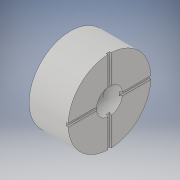
# Autodesk Inventor part: parabol_mirror_1_grooves
Saved by Autodesk Inventor 2019 (Build 230136000, 136)
## iProperties
Created: 2019-08-16
Part Number: parabol_mirror_1_grooves
Material: Generic
Document SubType Name: Modeling
Designer: CyrilLAPLANE
Density: 1 g/cm^3
Appearance: Default
Author: CyrilLAPLANE
Autodesk Inventor part; units mm, degrees
ref_plane "YZ Plane" through (0, 0, 0) normal (1, 0, 0) x (0, 1, 0)
ref_plane "XZ Plane" through (0, 0, 0) normal (0, 1, 0) x (-1, 0, 0)
ref_plane "XY Plane" through (0, 0, 0) normal (0, 0, 1) x (1, 0, 0)
sketch "Sketch2" plane through (0, 0, 0) normal (0, 0, 1) x (1, 0, 0)
  line L0 (1, 2) -> (1, 6.35)
  line L1 (1, 6.35) -> (-7.5, 6.35)
  line L2 (0, 0) -> (-5, 0)
  line L3 (-5, 0) -> (-5, 6.35)
  line L4 (-5, 6.35) -> (-7.5, 6.35)
  spline S0 degree 5 poles (0, 0) (-0.0014, 0.4587) (0.1367, 0.9206) (0.3862, 1.3172) (0.6748, 1.6754) (1, 2) knots 0 0 0 0 0 0 1 1 1 1 1 1
  line L5 (-5, 6.35) -> (1, 6.35)
  dimension "d13" = 5
  dimension "d18" = 6.35
  dimension "d19" = 2
  constraints: 12 end point, 1 collinear, 1 horizontal, 1 parallel, 1 perpendicular, 3 other
  measures "d13" distance of L2.start L2.end
  measures "d18" distance of L2.end L3.end
  measures "d19" vertical distance of L2.start L0.start
revolve "Revolution1" add sketch "Sketch2" angle 360 about axis through (0, 0, 0) along (-1, 0, 0)
sketch "Sketch4" plane through (1, 0, 0) normal (1, 0, 0) x (0, 0, -1)
  line L0 (-0.25, 12.7) -> (0.25, 12.7)
  line L1 (0.25, 12.7) -> (0.25, -12.7)
  line L2 (0.25, -12.7) -> (-0.25, -12.7)
  line L3 (-0.25, -12.7) -> (-0.25, 12.7)
  line L4 (12.7, -0.25) -> (-12.7, -0.25)
  line L5 (-12.7, -0.25) -> (-12.7, 0.25)
  line L6 (-12.7, 0.25) -> (12.7, 0.25)
  line L7 (12.7, 0.25) -> (12.7, -0.25)
  point P0 (0, 0)
  dimension "d34" = 0.5
  dimension "d35" = 0.25
  dimension "d36" = 12.7
  dimension "d37" = 12.7
  dimension "d38" = 0.5
  dimension "d39" = 0.25
  dimension "d40" = 12.7
  dimension "d41" = 12.7
  constraints: 16 end point, 4 parallel, 2 horizontal, 2 perpendicular
  measures "d34" distance between parallel lines of L3 L1
  measures "d35" distance from line of point (0, 0) L1
  measures "d36" distance from line of L2 point (0, 0)
  measures "d37" distance from line of L0 point (0, 0)
  measures "d38" distance of L4.end L5.end
  measures "d39" distance from line of L6 point (0, 0)
  measures "d40" distance from line of L5 point (0, 0)
  measures "d41" distance from line of L7 point (0, 0)
extrude "Extrusion2" cut sketch "Sketch4" against normal blind 0.25
equation "curve S0 of \"Sketch2\": x = t; y = (4*1*t)^(1/2); t from d10 to d11"
body "Solid1"
